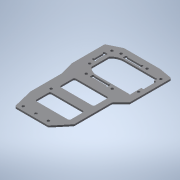
# Autodesk Inventor part: 胴体_サブフレーム_1_3
Saved by Autodesk Inventor 2020.4 (Build 244396000, 396)
## iProperties
Created: 2016-05-07
Part Number: 胴体_サブフレーム_1_3
Material: GFRP
Document SubType Name: Modeling
Designer: hiroaki
Density: 1.75 g/cm^3
Appearance: 滑らか - 淡い灰色
Mass: 16.1324 g
Surface Area: 112.711 cm^2
Volume: 9.21853 cm^3
Category: 胴体
d0: 1.000 ul
d2: 2.100 mm
d3: 2.000 mm
d4: 0.00 deg
Author: hiroaki
Autodesk Inventor part; units mm, degrees
ref_plane "YZ Plane" through (0, 0, 0) normal (1, 0, 0) x (0, 1, 0)
ref_plane "XZ Plane" through (0, 0, 0) normal (0, 1, 0) x (-1, 0, 0)
ref_plane "XY Plane" through (0, 0, 0) normal (0, 0, 1) x (1, 0, 0)
derived "胴体_基礎_1_3.ipt"
sketch "スケッチ1" plane through (0, 0, 0) normal (0, 0, 1) x (1, 0, 0)
  circle A0 centre (-15, 0) radius 1.55 projected
  circle A1 centre (15, 0) radius 1.55 projected
  line L0 (0, 0) -> (0, -11.5097) construction
  line L1 (-26, 56.6015) -> (-26, -5) projected
  line L2 (-26, -5) -> (28, -5) projected
  line L3 (-26, 56.6015) -> (-30.5, 73.218) projected
  line L4 (-30.5, 73.218) -> (-30.5, 112.7596) projected
  line L5 (-30.5, 112.7596) -> (-15, 120.25) projected
  line L6 (-15, 120.25) -> (28, 120.25) projected
  circle A2 centre (-3, 92) radius 11 construction
  line L7 (-15, 102.583) -> (-15, 81.417) construction
  line L8 (-3, 108) -> (36.5, 108) construction
  line L9 (36.5, 108) -> (36.5, 76) construction
  line L10 (36.5, 76) -> (-3, 76) construction
  arc A3 (-3, 108) -> (-15, 102.583) centre (-3, 92) ccw construction
  arc A4 (-15, 81.417) -> (-3, 76) centre (-3, 92) ccw construction
  line L11 (28, -5) -> (28, 73.75) projected
  line L12 (28, 73.75) -> (28, 120.25) construction
  line L13 (-2, 105.5) -> (25, 105.5) construction
  line L14 (25, 105.5) -> (25, 78.5) construction
  line L15 (25, 78.5) -> (-2, 78.5) construction
  line L16 (-2, 78.5) -> (-2, 105.5) construction
  circle A5 centre (-2, 105.5) radius 1.35 projected
  circle A6 centre (25, 105.5) radius 1.35 projected
  circle A7 centre (25, 78.5) radius 1.35 projected
  circle A8 centre (-2, 78.5) radius 1.35 projected
  circle A9 centre (-3, 92) radius 5.05 projected
  line L17 (-15, 110.25) -> (36.5, 110.25) construction
  line L18 (36.5, 110.25) -> (36.5, 73.75) construction
  line L19 (36.5, 73.75) -> (-15, 73.75) construction
  line L20 (-15, 73.75) -> (-15, 110.25) construction
  circle A10 centre (21.25, 92) radius 1.2 projected
  circle A11 centre (-3, 116.25) radius 1.2 projected
  circle A12 centre (-27.25, 92) radius 1.2 projected
  circle A13 centre (-3, 67.75) radius 1.2 projected
  line L21 (-6, 115.25) -> (15, 115.25) construction
  line L22 (15, 115.25) -> (15, 110.25) construction
  line L23 (15, 110.25) -> (-6, 110.25) construction
  line L24 (-6, 110.25) -> (-6, 115.25) construction
  circle A14 centre (-11, 112.75) radius 1.55 projected
  circle A15 centre (20, 112.75) radius 1.55 projected
  circle A16 centre (-11, 112.75) radius 7.5 construction
  circle A17 centre (-11, 71.25) radius 1.55 projected
  circle A18 centre (20, 71.25) radius 1.55 projected
  line L25 (-15, 92) -> (36.5, 92) construction
  line L26 (-6, 73.75) -> (15, 73.75) construction
  line L27 (15, 73.75) -> (15, 68.75) construction
  line L28 (15, 68.75) -> (-6, 68.75) construction
  line L29 (-6, 68.75) -> (-6, 73.75) construction
  line L30 (-15, 115.25) -> (24, 115.25) construction
  line L31 (24, 115.25) -> (24, 110.25) construction
  line L32 (24, 110.25) -> (-15, 110.25) construction
  line L33 (-15, 110.25) -> (-15, 115.25) construction
  circle A19 centre (-4.96, 112.84) radius 1.05
  circle A20 centre (-22, 50) radius 1.55 projected
  circle A21 centre (-22, 20) radius 1.55 projected
  circle A22 centre (-16.5, 34.75) radius 1.55 projected
  line L34 (-39.5, 5) -> (35.9852, 5) construction
  line L35 (35.9852, 5) -> (35.9852, -12.9857) construction
  line L36 (35.9852, -12.9857) -> (-39.5, -12.9857) construction
  line L37 (-39.5, -12.9857) -> (-39.5, 5) construction
  line L38 (-14, 60) -> (27, 60)
  line L39 (27, 60) -> (27, 42)
  line L40 (27, 42) -> (-14, 42)
  line L41 (-14, 42) -> (-14, 60)
  line L42 (-14, 31) -> (27, 31)
  line L43 (27, 31) -> (27, 13)
  line L44 (27, 13) -> (-14, 13)
  line L45 (-14, 13) -> (-14, 31)
  line L46 (-15.05, 102.6019) -> (-15.05, 81.3981)
  arc A23 (-15.05, 81.3981) -> (-3, 75.95) centre (-3, 92) ccw
  line L47 (-3, 75.95) -> (36.55, 75.95) construction
  line L48 (36.55, 75.95) -> (36.55, 108.05)
  line L49 (36.55, 108.05) -> (-3, 108.05) construction
  arc A24 (-3, 108.05) -> (-15.05, 102.6019) centre (-3, 92) ccw
  line L50 (28, 120.25) -> (28, 108.05)
  line L51 (28, 108.05) -> (-3, 108.05)
  line L52 (-3, 75.95) -> (28, 75.95)
  line L53 (28, 75.95) -> (28, 73.75)
  line L54 (-15.5, 120.25) -> (24.5, 120.25) construction
  line L55 (-6.01, 112.84) -> (15.01, 112.84)
  line L56 (15.01, 112.84) -> (15.01, 110.24)
  line L57 (15.01, 110.24) -> (-6.01, 110.24)
  line L58 (-6.01, 110.24) -> (-6.01, 112.84)
  circle A25 centre (-5.0584, 110.6837) radius 1.05
  line L59 (-6.01, 71.16) -> (15.01, 71.16)
  line L60 (15.01, 71.16) -> (15.01, 73.76)
  line L61 (15.01, 73.76) -> (-6.01, 73.76)
  line L62 (-6.01, 73.76) -> (-6.01, 71.16)
  circle A26 centre (-4.96, 71.16) radius 1.05
  circle A27 centre (13.96, 71.16) radius 1.05
  circle A28 centre (14.0584, 73.3163) radius 1.05
  circle A29 centre (-5.0584, 73.3163) radius 1.05
  circle A30 centre (-19.5, 105.25) radius 1.55 construction
  circle A31 centre (-19.5, 78.75) radius 1.55 construction
  line L63 (-22, 99.5) -> (-17, 99.5) construction
  line L64 (-17, 99.5) -> (-17, 84.5) construction
  line L65 (-17, 84.5) -> (-22, 84.5) construction
  line L66 (-22, 84.5) -> (-22, 99.5) construction
  circle A32 centre (-19.5, 100.55) radius 1.05 construction
  circle A33 centre (-26.5, 110.25) radius 1.55 projected
  circle A34 centre (-26.5, 73.75) radius 1.55 projected
  circle A35 centre (-26.5, 110.25) radius 4 construction
  circle A36 centre (-26.5, 73.75) radius 4 construction
  circle A37 centre (0, 0) radius 1.55 projected
  line L67 (15, 112.83) -> (-6, 112.83) construction
  line L68 (-6, 112.83) -> (-6, 110.25) construction
  line L69 (-6, 110.25) -> (15, 110.25) construction
  line L70 (15, 110.25) -> (15, 112.83) construction
  line L71 (-20, 5) -> (20, 5) projected
  line L72 (20, 5) -> (20, -5) projected
  line L73 (-20, 5) -> (-20, -5) projected
  line L74 (-20, -5) -> (-26, 19.5177) projected
  circle A38 centre (-22, 20) radius 4 projected
  line L75 (20, -5) -> (28, 4.534) projected
  line L76 (-15.05, 102.6019) -> (-14.1114, 102.1642) construction
  line L77 (-15.05, 102.6019) -> (-3, 108.05) construction
  circle A39 centre (-14.0984, 102.1581) radius 1.05
  circle A40 centre (-14.0984, 81.8419) radius 1.05
  circle A41 centre (-19.49, 83.75) radius 1.55
  circle A42 centre (-19.49, 110.25) radius 1.55
  circle A43 centre (-22, 103.47) radius 1.05
  circle A44 centre (-19.48, 103.48) radius 1.06
  circle A45 centre (-22, 90.55) radius 1.05
  circle A46 centre (-19.48, 90.55) radius 1.05
  line L78 (-22, 89.5) -> (-19.48, 89.5)
  line L79 (-22, 104.52) -> (-22, 89.5)
  line L80 (-19.48, 104.52) -> (-19.48, 89.5)
  circle A47 centre (14.0584, 110.6837) radius 1.05
  line L81 (-22, 104.52) -> (-19.48, 104.52)
  circle A48 centre (13.95, 112.83) radius 1.05
  point P0 (25, 92)
  point P1 (-6, 112.75)
  point P2 (-19.5, 99.5)
  point P3 (-26, 20)
  point P4 (-25.8853, 19.0492)
  point P5 (-6.01, 72.8725)
  point P6 (-4.1068, 73.76)
  point P7 (13.1068, 73.76)
  point P8 (15.01, 72.8725)
  point P9 (12.91, 71.16)
  point P10 (-3.91, 71.16)
  point P11 (-4.1068, 110.24)
  point P12 (-6.01, 111.1275)
  point P13 (-3.91, 112.84)
  point P14 (-14.6244, 80.9331)
  point P15 (-15.05, 82.2856)
  point P16 (-15.05, 101.7144)
  point P17 (-14.6244, 103.0669)
  point P18 (-19.48, 102.42)
  point P19 (-19.48, 91.6)
  point P20 (-19.48, 89.5)
  point P21 (-22, 91.6)
  point P22 (-22, 102.42)
  point P23 (-22, 104.52)
  point P24 (-6.01, 110.24)
  point P25 (-19.685, 104.52)
  point P26 (12.9, 112.84)
  point P27 (15, 112.84)
  point P28 (15.01, 111.1275)
  point P29 (13.1068, 110.24)
  dimension "d2" = 2.1
  dimension "d121" = 2.1
  dimension "d561" = 2.1
  dimension "d54" = 0.05
  dimension "d73" = 0.01
  dimension "d74" = 2.6
  dimension "d117" = 65
  dimension "d510" = 2.52
  dimension "d512" = 2.1
  dimension "d515" = 1
  dimension "d516" = 18
  dimension "d517" = 12
  dimension "d518" = 2.1
  dimension "d520" = 90
  dimension "d521" = 21.02
  dimension "d522" = 15.95
  dimension "d523" = 11
  dimension "d524" = 8
  dimension "d525" = 11.16
  dimension "d529" = 18.34
  dimension "d531" = 2.1
  dimension "d532" = 18.6837
  dimension "d534" = 51.55
  dimension "d535" = 22.4416
  dimension "d557" = 4.48
  dimension "d558" = 6.76
  dimension "d559" = 2.12
  dimension "d560" = 2.1
  dimension "d562" = 4.43
  dimension "d563" = 9.1519
  dimension "d568" = 15.02
  dimension "d569" = 7
  dimension "d570" = 9.2896
  dimension "d571" = 2.6837
  dimension "d572" = 14.4216
  dimension "d573" = 3.1
  dimension "d574" = 7.6481
  dimension "d575" = 2.51
  dimension "d576" = 3.1
  dimension "d577" = 4.44
  dimension "d578" = 6.8
  dimension "d579" = 11.0984
  dimension "d580" = 8.7081
  dimension "d581" = 2.6
  dimension "d582" = 21.02
  dimension "d584" = 2.1
  dimension "d585" = 2.1
  dimension "d586" = 2.1
  dimension "d587" = 2.1
  dimension "d589" = 2.19
  dimension "d590" = 9.04
  dimension "d591" = 13.48
  dimension "d592" = 4.79
  dimension "d594" = 2.1
  dimension "d595" = 2.6338
  dimension "d596" = 2.0584
  dimension "d597" = 11.16
  dimension "d598" = 11.16
  dimension "d599" = 14.04
  dimension "d600" = 2.6338
  dimension "d601" = 13.9416
  dimension "d602" = 26.01
  dimension "d603" = 4.78
  dimension "d604" = 14.05
  constraints: 70 end point, 15 centre point, 13 parallel, 8 point on line, 4 perpendicular, 4 point on circle, 3 collinear, 3 tangent, 2 horizontal, 1 vertical, 1 vertical alignment, 11 other
  measures "d54" radial gap between concentric circles of A24 A3
  measures "d73" distance between parallel lines of L57 L32
  measures "d74" distance of L57.end L55.start
  measures "d117" angle of L76 L46
  measures "d510" distance between parallel lines of L80 L79
  measures "d512" diameter of A46
  measures "d515" distance between parallel lines of L11 L39
  measures "d516" distance between parallel lines of L40 L38
  measures "d517" distance between parallel lines of L41 L1
  measures "d518" diameter of A25
  measures "d520" angle of L51 L58
  measures "d521" distance between parallel lines of L56 L58
  measures "d522" distance between parallel lines of L52 L38
  measures "d523" distance between parallel lines of L40 L42
  measures "d524" distance between parallel lines of L71 L44
  measures "d525" distance between parallel lines of L38 L59
  measures "d529" distance between parallel lines of L59 L78
  measures "d531" diameter of A47
  measures "d532" vertical distance of A9.centre A47.centre
  measures "d534" distance between parallel lines of L48 L7
  measures "d535" distance from line of L9 A47.centre
  measures "d557" distance from line of L20 A44.centre
  measures "d558" distance from line of L57 A44.centre
  measures "d559" diameter of A44
  measures "d560" diameter of A43
  measures "d562" distance from line of L46 A46.centre
  measures "d563" vertical distance of L46.end A46.centre
  measures "d568" distance between parallel lines of L78 L81
  measures "d569" distance from line of L20 A43.centre
  measures "d570" vertical distance of L4.end A43.centre
  measures "d571" vertical distance of L8.start A25.centre
  measures "d572" horizontal distance of A44.centre A25.centre
  measures "d573" diameter of A42
  measures "d574" vertical distance of L46.start A42.centre
  measures "d575" horizontal distance of A42.centre A43.centre
  measures "d576" diameter of A41
  measures "d577" distance from line of L46 A41.centre
  measures "d578" distance of A46.centre A41.centre
  measures "d579" horizontal distance of A9.centre A40.centre
  measures "d580" vertical distance of A46.centre A40.centre
  measures "d581" distance of L61.end L62.end
  measures "d582" distance of L59.start L59.end
  measures "d584" diameter of A29
  measures "d585" diameter of A26
  measures "d586" diameter of A28
  measures "d587" diameter of A27
  measures "d589" distance between parallel lines of L61 L52
  measures "d590" distance between parallel lines of L62 L46
  measures "d591" distance from line of A42.centre L58
  measures "d592" distance from line of L49.end L55
  measures "d594" diameter of A48
  measures "d595" vertical distance of L47.start A29.centre
  measures "d596" horizontal distance of L47.start A29.centre
  measures "d597" distance from line of L38 A26.centre
  measures "d598" distance from line of L38 A27.centre
  measures "d599" distance from line of L12 A27.centre
  measures "d600" distance from line of L52 A28.centre
  measures "d601" distance from line of L12 A28.centre
  measures "d602" distance from line of A17.centre L60
  measures "d603" distance from line of L51 A48.centre
  measures "d604" distance from line of L50 A48.centre
extrude "押し出し1" add sketch "スケッチ1" along normal blind 2 contours L1 L3 L4 L5 L6 L50 L51 A24 A39 L46 A40 A23 L52 L53 L11 L75 L72 L71 L73 L74 A38 | A38 | L73 L71 L72 L2 | A11 | A12 | A13 | A20 | A21 | A33 | A34
sketch "スケッチ5" plane through (-15, 120.25, 2) normal (0, 0, 1) x (1, 0, 0)
  line L0 (-0.05, -37.9644) -> (-0.05, -18.5356)
  line L1 (43, -12.2) -> (43, 0)
  line L2 (43, 0) -> (59.5, -2.9094)
  line L3 (59.5, -2.9094) -> (59.5, -52.9094)
  line L4 (43, -44.3) -> (50.0151, -44.3)
  line L5 (50.0151, -12.2) -> (43, -12.2)
  line L6 (54.01, -20.74) -> (54.01, -22.2249) construction
  line L7 (12, -28.25) -> (-0.05, -28.25) construction
  arc A0 (51.5, -13.6849) -> (50.0151, -12.2) centre (50.7575, -12.9425) ccw
  line L8 (51.5, -13.6849) -> (51.5, -12.2) construction
  line L9 (51.5, -12.2) -> (50.0151, -12.2) construction
  arc A1 (50.0151, -44.3) -> (51.5, -42.8151) centre (50.7575, -43.5575) ccw
  line L10 (51.5, -42.8151) -> (51.5, -44.3) construction
  line L11 (50.0151, -44.3) -> (51.5, -44.3) construction
  line L12 (59.5, -52.9094) -> (49, -63.4094)
  line L13 (49, -63.4094) -> (49, -108.5654)
  line L14 (35, -125.25) -> (43, -115.716) projected
  line L15 (43, -115.716) -> (49, -108.5654)
  line L16 (35, -125.25) -> (43, -115.716) projected
  line L17 (52.5251, -15.7395) -> (51.5, -15.7395)
  line L18 (52.5257, -30.76) -> (52.5257, -30.76)
  line L19 (52.5257, -30.76) -> (51.5, -30.76)
  line L20 (54.01, -17.2245) -> (54.01, -29.2745)
  arc A2 (54.01, -17.2245) -> (52.5251, -15.7395) centre (53.2675, -16.482) ccw
  line L21 (51.5, -30.76) -> (51.5, -42.8151)
  line L22 (51.5, -13.6849) -> (51.5, -15.7395)
  circle A3 centre (54, -10) radius 1.55
  circle A4 centre (54, -36.5) radius 1.55
  line L23 (-0.05, -37.9644) -> (-0.05, -18.5356) projected
  line L24 (43, -115.716) -> (43, -44.3) projected
  line L25 (43, -44.3) -> (12, -44.3) projected
  line L26 (43, 0) -> (0, 0) projected
  circle A5 centre (50.7575, -12.9425) radius 1.05 construction
  arc A6 (52.5257, -30.76) -> (54.01, -29.2745) centre (53.2678, -30.0172) ccw
  point P0 (15, -120.25)
  point P1 (51.5, -13.6849)
  point P2 (51.5, -42.8151)
  point P3 (52.5251, -15.7395)
  point P4 (54.01, -17.2245)
  dimension "d104" = 45
  dimension "d106" = 50
  dimension "d125" = 12.05
  dimension "d129" = 12.0551
  dimension "d130" = 2.0546
  dimension "d438" = 8.5
  dimension "d440" = 11.01
  dimension "d441" = 1.0251
  dimension "d498" = 6
  dimension "d499" = 16.5
  dimension "d538" = 1.05
  dimension "d539" = 3.1
  dimension "d540" = 13.54
  dimension "d543" = 0.7425
  dimension "d544" = 3.5395
  dimension "d545" = 11
  dimension "d546" = 10
  dimension "d547" = 7.8
  dimension "d548" = 5.5
  dimension "d549" = 3.1
  dimension "d550" = 12.9425
  dimension "d554" = 17.8172
  dimension "d555" = 1.05
  dimension "d556" = 10.2678
  constraints: 41 end point, 8 point on circle, 7 centre point, 5 parallel, 4 collinear, 2 horizontal, 2 vertical, 1 coincident, 1 concentric, 1 midpoint, 1 perpendicular, 3 other
  measures "d104" angle of L12 L4
  measures "d106" distance of L2.end L3.end
  measures "d125" distance of L20.start L20.end
  measures "d129" distance of L19.end L21.end
  measures "d130" distance of L22.start L17.end
  measures "d438" distance from line of L22 L1.start
  measures "d440" distance from line of L20 L1.start
  measures "d441" distance of L17.start L17.end
  measures "d498" distance between parallel lines of L13 L24
  measures "d499" distance from line of L3.end L24
  measures "d538" radius of A0
  measures "d539" diameter of A3
  measures "d540" distance between parallel lines of L4 L19
  measures "d543" distance from line of L22 A0.centre
  measures "d544" distance between parallel lines of L5 L17
  measures "d545" distance from line of A3.centre L1
  measures "d546" distance from line of L26 A3.centre
  measures "d547" vertical distance of L4.start A4.centre
  measures "d548" distance from line of L3 A4.centre
  measures "d549" diameter of A4
  measures "d550" distance from line of A0.centre L26
  measures "d554" vertical distance of L1.start A6.centre
  measures "d555" radius of A6
  measures "d556" horizontal distance of L4.start A6.centre
extrude "押し出し6" add sketch "スケッチ5" against normal blind 2
fillet "フィレット5" radius 2 19 edges at (27, 42, 1) (27, 60, 1) (-14, 60, 1) (-14, 42, 1) (27, 13, 1) (27, 31, 1) (-14, 31, 1) (-14, 13, 1) (-30.5, 112.7596, 1) (-15, 120.25, 1) (28, 120.25, 1) (44.5, 117.3406, 1) (44.5, 67.3406, 1) (34, 56.8406, 1) (34, 11.6846, 1) (20, -5, 1) (-30.5, 73.218, 1) (-26, 56.6015, 1) (-20, -5, 1)
